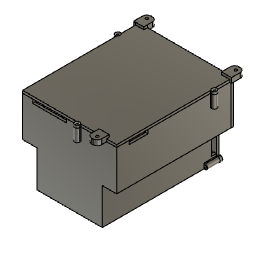
Caja de Circuitos PLA (Autodesk Fusion 360 design; units mm, degrees)
Autodesk Fusion 360 part; units mm, degrees
note: some values were not read from the file. Set by a fixed rule: which sketch regions a step uses.
(part 1 of 2)
sketch "Sketch1" plane through (0, 0, 0) normal (0, 1, 0) x (1, 0, 0)
  line L0 (-24, -14.5) -> (-24, 14.5)
  line L1 (-24, 14.5) -> (24, 14.5)
  line L2 (24, 14.5) -> (24, -14.5)
  line L3 (24, -14.5) -> (-24, 14.5) construction
  line L4 (-24, -14.5) -> (24, 14.5) construction
  line L5 (-24, -14.5) -> (-24, -44.5) construction
  line L6 (-35.5, -44.5) -> (35.5, -44.5) construction
  line L7 (35.5, -44.5) -> (35.5, -14.5)
  line L8 (24, -14.5) -> (-24, -14.5) construction
  line L9 (-35.5, -14.5) -> (-35.5, -44.5)
  line L10 (-35.5, -44.5) -> (35.5, -14.5) construction
  line L11 (35.5, -44.5) -> (-35.5, -14.5) construction
  line L12 (-24, -14.5) -> (-35.5, -14.5)
  line L13 (35.5, -14.5) -> (24, -14.5)
  line L14 (37.5, -44.5) -> (37.5, -12.5)
  line L15 (37.5, -12.5) -> (26, -12.5)
  line L16 (26, 16.5) -> (26, -12.5)
  line L17 (-26, 16.5) -> (26, 16.5)
  line L18 (-26, -12.5) -> (-26, 16.5)
  line L19 (-26, -12.5) -> (-37.5, -12.5)
  line L20 (-37.5, -12.5) -> (-37.5, -44.5)
  line L21 (-37.5, -44.5) -> (-35.5, -44.5)
  line L22 (35.5, -44.5) -> (37.5, -44.5)
  point P0 (0, -29.5)
  dimension "d1" = 48
  dimension "d4" = 29
  dimension "d5" = 30
  dimension "d6" = 71
  dimension "d7" = -2
  constraint parallel L0 L2
  constraint coincident L3 origin
  constraint coincident L4 origin
  constraint horizontal L6
  constraint perpendicular L6 L7
  constraint parallel L6 L8
  constraint parallel L7 L9
  constraint coincident L10 P0
  constraint coincident L11 P0
  constraint parallel L6 L12
  constraint parallel L6 L13
  constraint perpendicular L9 L21
  measures "d1" distance of L0.end L1.end
  measures "d4" distance of L0.start L0.end
  measures "d5" distance of L0.start L5.end
  measures "d6" distance of L7.end L9.start
extrude "Extrude1" add sketch "Sketch1" along normal blind 89 makes body 1
ref_plane "WorkPlane1" through (0, 0, 14) normal (0, -1, 0) x (-1, 0, 0)
sketch "Sketch2" plane through (0, 0, 14) normal (0, -1, 0) x (1, 0, 0)
  line L0 (-37.5, -1.5) -> (-37.5, 30.5)
  line L1 (-26, -1.5) -> (-37.5, -1.5)
  line L2 (-26, -1.5) -> (-26, -30.5)
  line L3 (-26, -30.5) -> (26, -30.5)
  line L4 (26, -30.5) -> (26, -1.5)
  line L5 (37.5, -1.5) -> (26, -1.5)
  line L6 (37.5, 30.5) -> (37.5, -1.5)
  line L7 (-37.5, 30.5) -> (37.5, 30.5)
  constraint coincident L0.end L7.start
  constraint coincident L6.start L7.end
extrude "Extrude2" add sketch "Sketch2" along normal blind 2 bodies 1
ref_plane "WorkPlane2" through (0, 89, 14) normal (0, 1, 0) x (0, 0, 1)
sketch "Sketch3" plane through (0, 89, 14) normal (0, 1, 0) x (1, 0, 0)
  line L0 (-26, 1.5) -> (-26, 30.5)
  line L1 (-26, 30.5) -> (26, 30.5)
  line L2 (26, 30.5) -> (26, 1.5)
  line L3 (26, 1.5) -> (37.5, 1.5)
  line L4 (37.5, 1.5) -> (37.5, -30.5)
  line L5 (37.5, -30.5) -> (-37.5, -30.5)
  line L6 (-37.5, -30.5) -> (-37.5, 1.5)
  line L7 (-37.5, 1.5) -> (-26, 1.5)
extrude "Extrude3" add sketch "Sketch3" along normal blind 2 separate body makes body 2
ref_plane "WorkPlane3" through (0, 43.5, 44.5) normal (0, 0, 1) x (1, 0, 0)
sketch "Sketch4" plane through (0, 43.5, 44.5) normal (0, 0, 1) x (1, 0, 0)
  line L0 (-37.5, 47.5) -> (37.5, 47.5)
  line L1 (-37.5, -45.5) -> (-37.5, 45.5)
  line L2 (37.5, -45.5) -> (-37.5, -45.5)
  line L3 (37.5, -45.5) -> (37.5, 45.5)
  line L4 (-37.5, 45.5) -> (-37.5, 47.5)
  line L5 (37.5, 45.5) -> (37.5, 47.5)
extrude "Extrude4" add sketch "Sketch4" along normal blind 2 bodies 2
ref_plane "WorkPlane4" through (37.5, 43.5, 28.5) normal (1, 0, 0) x (0, 0, -1)
sketch "Sketch5" plane through (37.5, 43.5, 28.5) normal (1, 0, 0) x (0, 1, 0)
  line L0 (-45.5, 16) -> (-35.5, 16) construction
  line L1 (-35.5, 17.9292) -> (-20.5, 17.9292)
  line L2 (-35.5, 16) -> (-20.5, 16)
  line L3 (-20.5, 16) -> (-20.5, 13)
  line L4 (-20.5, 13) -> (-35.5, 13)
  line L5 (-35.5, 13) -> (-35.5, 16)
  point P0 (-45.5, 16)
  dimension "d20" = 10
  dimension "d21" = 15
  dimension "d22" = 3
  constraint coincident P0 L0.start
  constraint horizontal L0
  constraint parallel L0 L1
  constraint horizontal L2
  constraint vertical L3
  constraint horizontal L4
  constraint vertical L5
  measures "d20" distance of P0 L0.end
  measures "d21" distance of L1.start L1.end
  measures "d22" distance of L0.end L4.end
extrude "Extrude5" cut sketch "Sketch5" against normal blind 85 bodies 1
ref_plane "WorkPlane5" through (0, -2, 14) normal (0, -1, 0) x (0, 0, -1)
sketch "Sketch6" plane through (0, -2, 14) normal (0, -1, 0) x (1, 0, 0)
  line L0 (-37.5, 30.5) -> (-29.5, 30.5)
  line L1 (-29.5, 33.204) -> (-2.5, 33.204)
  line L2 (-29.5, 30.5) -> (-2.5, 30.5)
  line L3 (-2.5, 30.5) -> (-2.5, 27.5)
  line L4 (-2.5, 27.5) -> (-29.5, 27.5)
  line L5 (-29.5, 27.5) -> (-29.5, 30.5)
  point P0 (-37.5, 30.5)
  dimension "d26" = 8
  dimension "d27" = 27
  dimension "d28" = 3
  constraint coincident P0 L0.start
  constraint horizontal L0
  constraint parallel L0 L1
  constraint horizontal L2
  constraint vertical L3
  constraint horizontal L4
  constraint vertical L5
  measures "d26" distance of P0 L0.end
  measures "d27" distance of L1.start L1.end
  measures "d28" distance of L0.end L4.end
extrude "Extrude6" cut sketch "Sketch6" against normal blind 10 bodies 1
ref_plane "WorkPlane6" through (0, 43.5, 44.5) normal (0, 0, -1) x (-1, 0, 0)
sketch "Sketch7" plane through (0, 43.5, 44.5) normal (0, 0, -1) x (1, 0, 0)
  line L0 (-37.5, -45.5) -> (37.5, -45.5)
  line L1 (37.5, -45.5) -> (37.5, 45.5)
  line L2 (37.5, 45.5) -> (-37.5, 45.5)
  line L3 (-37.5, 45.5) -> (-37.5, -45.5)
  line L4 (-35.5, -43.5) -> (35.5, -43.5)
  line L5 (35.5, -43.5) -> (35.5, 43.5)
  line L6 (35.5, 43.5) -> (-35.5, 43.5)
  line L7 (-35.5, 43.5) -> (-35.5, -43.5)
  line L8 (-33.5, -41.5) -> (33.5, -41.5)
  line L9 (33.5, -41.5) -> (33.5, 41.5)
  line L10 (33.5, 41.5) -> (-33.5, 41.5)
  line L11 (-33.5, 41.5) -> (-33.5, -41.5)
  line L12 (-29.5, 45.5) -> (-29.5, 41.5)
  line L13 (-2.5, 45.5) -> (-2.5, 41.5)
  line L14 (37.5, 35.5) -> (-35.5, 35.5)
  line L15 (37.5, 20.5) -> (-35.5, 20.5)
  line L16 (-35.5, -41.5) -> (35.5, -41.5)
  point P0 (-29.5, 45.5)
  point P1 (-2.5, 45.5)
  point P2 (37.5, 35.5)
  point P3 (37.5, 20.5)
  dimension "d32" = -2
  dimension "d33" = -4
  constraint coincident P0 L12.start
  constraint coincident L10 L12.end
  constraint perpendicular L10 L12
  constraint coincident P1 L13.start
  constraint coincident L10 L13.end
  constraint perpendicular L10 L13
  constraint coincident P2 L14.start
  constraint coincident L7 L14.end
  constraint perpendicular L7 L14
  constraint coincident P3 L15.start
  constraint coincident L7 L15.end
  constraint perpendicular L7 L15
  constraint coincident L7 L16.start
  constraint coincident L5 L16.end
  constraint perpendicular L5 L16
extrude "Extrude7" add sketch "Sketch7" along normal blind 2 contours L5 L9 L15 L16 | L6 L7 L10 L11 L12 L14 | L5 L6 L9 L10 L13 L14 | L7 L11 L15 L16 bodies 2
ref_plane "WorkPlane7" through (0, 89, 14) normal (0, -1, 0) x (-1, 0, 0)
sketch "Sketch8" plane through (0, 89, 14) normal (0, -1, 0) x (1, 0, 0)
  line L0 (-37.5, 30.5) -> (-37.5, -1.5)
  line L1 (-37.5, -1.5) -> (-26, -1.5)
  line L2 (-26, -1.5) -> (-26, -30.5)
  line L3 (-26, -30.5) -> (26, -30.5)
  line L4 (26, -30.5) -> (26, -1.5)
  line L5 (26, -1.5) -> (37.5, -1.5)
  line L6 (37.5, -1.5) -> (37.5, 30.5)
  line L7 (-35.5, 30.5) -> (-35.5, 0.5)
  line L8 (-35.5, 0.5) -> (-24, 0.5)
  line L9 (-24, 0.5) -> (-24, -28.5)
  line L10 (-24, -28.5) -> (24, -28.5)
  line L11 (24, -28.5) -> (24, 0.5)
  line L12 (24, 0.5) -> (35.5, 0.5)
  line L13 (35.5, 0.5) -> (35.5, 30.5)
  line L14 (-33.5, 30.5) -> (-33.5, 2.5)
  line L15 (-33.5, 2.5) -> (-22, 2.5)
  line L16 (-22, 2.5) -> (-22, -26.5)
  line L17 (-22, -26.5) -> (22, -26.5)
  line L18 (22, -26.5) -> (22, 2.5)
  line L19 (22, 2.5) -> (33.5, 2.5)
  line L20 (33.5, 2.5) -> (33.5, 30.5)
  line L21 (-35.5, 30.5) -> (35.5, 30.5)
  dimension "d37" = -2
  dimension "d38" = -4
  constraint perpendicular L13 L21
extrude "Extrude8" add sketch "Sketch8" along normal blind 2 contours L7 L8 L9 L10 L11 L12 L13 L14 L15 L16 L17 L18 L19 L20 L21 bodies 2
ref_plane "WorkPlane8" through (0, 44.5, 46.5) normal (0, 0, 1) x (1, 0, 0)
sketch "Sketch9" plane through (0, 44.5, 46.5) normal (0, 0, 1) x (1, 0, 0)
  circle A0 centre (7.0001, -47.5) radius 1
  line L0 (8.9999, -46.5) -> (11.0001, -46.5)
  line L1 (8.9999, -46.5) -> (9.0001, -47.4997)
  arc A1 (5.0001, -47.5) -> (9.0001, -47.4997) centre (7.0001, -47.5) ccw
  line L2 (5.0001, -47.5) -> (5.0001, -46.5)
  line L3 (5.0001, -46.5) -> (3.0001, -46.5)
  line L4 (-37.5, -46.5) -> (37.5, -46.5)
  line L5 (35.5, -44.5) -> (-2.5, -44.5)
  line L6 (16.5, -44.5) -> (16.5, -51.9184)
  line L7 (16.5, -51.9184) -> (-2.5, -51.9184)
  line L8 (16.5, -44.5) -> (35.5, -44.5)
  line L9 (26, -44.5) -> (26, -35)
  line L10 (5.0001, -46.5) -> (8.9999, -46.5)
  line L11 (37.5, -21.5) -> (37.5, -36.5)
  line L12 (-37.5, 46.5) -> (-37.5, -46.5)
  line L13 (37.5, -46.5) -> (37.5, 46.5)
  line L14 (37.5, 46.5) -> (-37.5, 46.5)
  line L15 (-37.5, 46.5) -> (-37.5, -46.5)
  line L16 (-37.5, -46.5) -> (37.5, -46.5)
  line L17 (40, -10) -> (-40, -10)
  line L18 (37.5, 32.2975) -> (38.4997, 32.2977)
  arc A2 (38.5, 28.2977) -> (38.4997, 32.2977) centre (38.5, 30.2977) ccw
  line L19 (37.5, 32.2975) -> (37.5, 24.2977)
  line L20 (38.5, 28.2977) -> (37.5, 28.2977)
  circle A3 centre (38.5, 30.2977) radius 1
  line L21 (37.5, 28.2977) -> (37.5, 32.2975)
  line L22 (-38.5, 32.2975) -> (-37.5, 32.2975)
  circle A4 centre (-38.5, 30.2975) radius 1
  arc A5 (-38.5, 32.2975) -> (-38.4997, 28.2975) centre (-38.5, 30.2975) ccw
  line L23 (-37.5, 32.2975) -> (-37.5, 28.2977)
  line L24 (-37.5, 28.2977) -> (-38.4997, 28.2975)
  line L25 (-37.5, 28.2977) -> (-37.5, 16.2975)
  line L26 (37.5, 46.5) -> (33.5003, 46.5)
  line L27 (-33.5003, 46.5) -> (-37.5, 46.5)
  line L28 (-37.5, 30.2976) -> (37.5, 30.2976)
  line L29 (35.4998, 50.5) -> (35.4998, 49.5)
  circle A6 centre (35.4998, 50.5) radius 1
  line L30 (33.4997, 50.5) -> (33.4997, 50.4997)
  arc A7 (33.4997, 50.5) -> (33.4997, 50.4993) centre (35.4998, 50.5) ccw
  arc A8 (38.9998, 50.5) -> (34.9998, 53.9641) centre (35.4998, 50.5) ccw
  line L31 (38.4998, 43.5) -> (37.5, 43.5)
  line L32 (37.5, 46.5) -> (37.5, 43.5)
  line L33 (30.9998, 50.5) -> (30.9998, 46.5)
  line L34 (34.2365, 53.9901) -> (35.7632, 53.9901)
  line L35 (38.9998, 50.5) -> (38.9998, 43.5)
  line L36 (38.9998, 43.5) -> (37.5, 43.5)
  arc A9 (34.9998, 53.9641) -> (30.9998, 50.5) centre (34.4998, 50.5) ccw
  line L37 (0, 46.5) -> (0, 51.2854)
  circle A10 centre (-35.4998, 50.5) radius 1
  line L38 (-33.4997, 50.5) -> (-33.4997, 50.4997)
  line L39 (-30.9998, 50.5) -> (-30.9998, 46.5)
  arc A11 (-34.9998, 53.9641) -> (-38.9998, 50.5) centre (-35.4998, 50.5) ccw
  line L40 (-38.9998, 50.5) -> (-38.9998, 43.5)
  arc A12 (-30.9998, 50.5) -> (-34.9998, 53.9641) centre (-34.4998, 50.5) ccw
  line L41 (-34.2365, 53.9901) -> (-35.7632, 53.9901)
  line L42 (-37.5, 46.5) -> (-33.5003, 46.5)
  line L43 (-37.5, 46.5) -> (-37.5, 43.5)
  line L44 (-35.4998, 50.5) -> (-35.4998, 49.5)
  line L45 (-38.9998, 43.5) -> (-37.5, 43.5)
  arc A13 (-33.4997, 50.4993) -> (-33.4997, 50.5) centre (-35.4998, 50.5) ccw
  line L46 (-38.4998, 43.5) -> (-37.5, 43.5)
  line L47 (26, -49.5) -> (26, -50.5)
  circle A14 centre (26, -50.5) radius 1
  line L48 (21.5, -50.5) -> (21.5, -46.5)
  line L49 (29.5, -50.5) -> (29.5, -46.5)
  line L50 (24.7991, -53.9942) -> (26.1016, -53.9985)
  arc A15 (21.5, -50.5) -> (25.1779, -53.9955) centre (25, -50.5) ccw
  arc A16 (25.9998, -50.5) -> (26, -50.5) centre (26.0002, -48.5) ccw
  arc A17 (25.8753, -53.9978) -> (29.5, -50.5) centre (26, -50.5) ccw
  line L51 (21.5, -46.5) -> (29.5, -46.5)
  point P0 (7.0001, -47.5)
  point P1 (7, -46.5)
  point P2 (26, -46.5)
  point P3 (26.0002, -48.5)
  point P4 (7, -46.5)
  point P5 (37.5, -21.5)
  point P6 (38.5, 30.2977)
  point P7 (37.5, 30.2976)
  point P8 (37.5, 30.2976)
  point P9 (-37.5, 30.2976)
  point P10 (-38.5, 30.2975)
  point P11 (-37.5, 30.2976)
  point P12 (35.5, 48.5)
  point P13 (-37.5, 46.5)
  point P14 (-35.5, 48.5)
  dimension "d42" = 2
  dimension "d2" = 4
  dimension "d48" = 2
  dimension "d49" = 4
  dimension "d50" = 2
  dimension "d51" = 4
  dimension "d128" = 7
  dimension "d129" = 2
  dimension "d135" = 4.5
  constraint coincident A0.centre A1.centre
  constraint concentric A0 A1
  constraint tangent A0 L0
  constraint horizontal L0
  constraint tangent A0 L3
  constraint perpendicular L2 L3
  constraint coincident L1.end A1
  constraint tangent L1 A1
  constraint coincident A1.end L1
  constraint midpoint L5 L6.start
  constraint perpendicular L4 L6
  constraint perpendicular L6 L7
  constraint coincident L5.start L8.end
  constraint midpoint L8 L9.start
  constraint perpendicular L5 L9
  constraint coincident L4 P4
  constraint coincident L4 P2
  constraint parallel L0 L10
  constraint midpoint L10 P4
  constraint perpendicular L15 L17
  constraint coincident P6 A2.centre
  constraint concentric A2 A3
  constraint tangent L19 A3
  constraint coincident L18.end A2
  constraint tangent L18 A2
  constraint coincident A2.end L18
  constraint parallel L19 L21
  constraint midpoint P8 L21
  constraint coincident P10 A4.centre
  constraint concentric A4 A5
  constraint tangent A4 L25
  constraint coincident L24.end A5
  constraint tangent A5 L24
  constraint coincident A5.end L24
  constraint parallel L23 L25
  constraint midpoint P11 L23
  constraint coincident P11 P9
  constraint coincident L13 P8
  constraint perpendicular L13 L28
  constraint vertical L29
  constraint coincident L29.start A6.centre
  constraint concentric A6 A8
  constraint concentric A7 A8
  constraint coincident L13.end L14.start
  constraint coincident L30 A7.end
  constraint coincident L13 L31.end
  constraint perpendicular L13 L31
  constraint coincident L14 L33.end
  constraint perpendicular L14 L33
  constraint coincident A8 L34.end
  constraint perpendicular L33 L34
  constraint tangent A8 L35
  constraint perpendicular L32 L36
  constraint coincident A7 L30.end
  constraint midpoint L14 L37.start
  constraint perpendicular L14 L37
  constraint symmetric L13.end L37 P13
  constraint symmetric P12 L37 P14
  constraint symmetric L26.end L37 L27.start
  constraint symmetric L29.start L37 A10.centre
  constraint symmetric L29.end L37 L44.end
  constraint symmetric A6 L37 A10
  constraint symmetric L30.start L37 L38.start
  constraint symmetric A7 L37 A13
  constraint symmetric A8 L37 A11
  constraint symmetric A7.end L37 A13.start
  constraint symmetric L31.start L37 L46.start
  constraint symmetric L31.end L37 L43.end
  constraint symmetric L33.start L37 L39.start
  constraint symmetric L33.end L37 L39.end
  constraint symmetric L34.start L37 L41.start
  constraint symmetric L34.end L37 L41.end
  constraint symmetric A8.start L37 A11.end
  constraint symmetric L35.end L37 L40.end
  constraint symmetric A9 L37 A12
  constraint symmetric A8.end L37 A11.start
  constraint symmetric L30.end L37 L38.end
  constraint perpendicular L16 L47
  constraint coincident L47.end A14.centre
  constraint concentric A14 A17
  constraint coincident A14 A15.centre
  constraint coincident L4 L48.end
  constraint tangent L48 A15
  constraint coincident L16 L49.end
  constraint tangent L49 A17
  constraint perpendicular L16 L49
  constraint coincident L50.start A15
  constraint coincident L50.end A17
  constraint coincident L50 A15.end
  constraint coincident L50 A17.start
  constraint coincident A14 L47.start
  constraint perpendicular L48 L51
  measures "d42" diameter of A0
  measures "d2" diameter of A1
  measures "d48" diameter of A3
  measures "d49" diameter of A2
  measures "d50" diameter of A4
  measures "d51" diameter of A5
  measures "d128" diameter of A8
  measures "d129" diameter of A6
  measures "d135" distance of L47.end L48.start
extrude "Extrude9" add sketch "Sketch9" against normal blind 2 contours L1 A1 L2 L4 L10 L16 | L12 L15 L22 A5 L23 L24 | L13 L18 A2 L19 L20 L21 bodies 2
ref_plane "WorkPlane9" through (0, 43.5, 44.5) normal (0, 0, 1) x (1, 0, 0)
sketch "Sketch10" plane through (17.5, 3, 44.5) normal (0, 0, 1) x (1, 0, 0)
  circle A0 centre (-56, 71.7975) radius 1
  circle A1 centre (-10.4999, -6) radius 1
  line L0 (-55, 73.7975) -> (-56, 73.7975)
  arc A2 (-56, 73.7975) -> (-55.9997, 69.7975) centre (-56, 71.7975) ccw
  line L1 (-55.9997, 69.7975) -> (-55, 69.7977)
  line L2 (-55, 88) -> (-55, 73.7975)
  line L3 (-8.5001, -5) -> (20, -5)
  line L4 (-12.4999, -5) -> (-12.4999, -6)
  arc A3 (-12.4999, -6) -> (-8.4999, -5.9997) centre (-10.4999, -6) ccw
  line L5 (-8.4999, -5.9997) -> (-8.5001, -5)
  line L6 (20, 73.7975) -> (20, 88)
  line L7 (20, 88) -> (-55, 88)
  line L8 (-12.4999, -5) -> (-8.5001, -5)
  line L9 (-55, 88) -> (-55, 73.7975)
  circle A4 centre (21, 71.7977) radius 1
  line L10 (20, 69.7977) -> (21, 69.7977)
  arc A5 (21, 69.7977) -> (20.9997, 73.7977) centre (21, 71.7977) ccw
  line L11 (20.9997, 73.7977) -> (20, 73.7975)
  line L12 (20, -5) -> (20, 69.7977)
  line L13 (20, 73.7975) -> (20, 69.7977)
  line L14 (20, 73.7975) -> (20, 69.7977)
  line L15 (-55, 69.7977) -> (-55, -5)
  line L16 (-55, -5) -> (-12.4999, -5)
  constraint coincident L4.start L8.start
  constraint coincident L3.start L5.end
  constraint coincident L2.start L7.end
  constraint coincident L0.start L2.end
  constraint coincident L6.start L11.end
  constraint coincident L10.start L12.end
extrude "Extrude11" add sketch "Sketch10" against normal blind 10 bodies 1
fillet "Fillet1" radius 0.95 3 edges at (6.0678, -3.3616, 46.5) (37.5677, 74.4361, 46.5) (-39.4323, 74.4359, 46.5) on bodies 2
ref_plane "WorkPlane10" through (0, 91, 15) normal (0, 1, 0) x (0, 0, 1)
sketch "Sketch11" plane through (0, 91, 15) normal (0, 1, 0) x (1, 0, 0)
  line L0 (26, 31.5) -> (26, 33.5002)
  line L1 (26, 27.5002) -> (26, 25.5002)
  line L2 (26, 31.5) -> (26.9997, 31.5002)
  circle A0 centre (27, 29.5002) radius 1
  line L3 (27, 27.5002) -> (26, 27.5002)
  arc A1 (27, 27.5002) -> (26.9997, 31.5002) centre (27, 29.5002) ccw
  line L4 (-26, 27.5002) -> (-26, 25.5)
  line L5 (-26, 31.5) -> (-26, 33.5)
  line L6 (-26, 27.5002) -> (-26.9997, 27.5)
  arc A2 (-27, 31.5) -> (-26.9997, 27.5) centre (-27, 29.5) ccw
  circle A3 centre (-27, 29.5) radius 1
  line L7 (-27, 31.5) -> (-26, 31.5)
  line L8 (37.5, -31.5) -> (37.5, 2.5)
  line L9 (37.5, 2.5) -> (26, 2.5)
  line L10 (26, 2.5) -> (26, 31.5)
  line L11 (26, 31.5) -> (-26, 31.5)
  line L12 (-26, 31.5) -> (-26, 2.5)
  line L13 (-26, 2.5) -> (-37.5, 2.5)
  line L14 (-37.5, 2.5) -> (-37.5, -31.5)
  line L15 (-37.5, -31.5) -> (37.5, -31.5)
  line L16 (26, 27.5002) -> (26, 31.5)
  line L17 (-26, 27.5002) -> (-26, 31.5)
  point P0 (27, 29.5002)
  point P1 (-27, 29.5)
  dimension "d64" = 2
  dimension "d65" = 4
  dimension "d66" = 2
  dimension "d67" = 4
  constraint coincident P0 A0.centre
  constraint concentric A0 A1
  constraint tangent L0 A0
  constraint tangent L1 A0
  constraint perpendicular L1 L3
  constraint coincident L2.end A1
  constraint tangent L2 A1
  constraint coincident A1.end L2
  constraint coincident P1 A2.centre
  constraint concentric A2 A3
  constraint tangent L4 A3
  constraint tangent L5 A3
  constraint perpendicular L5 L7
  constraint coincident L6.end A2
  constraint tangent L6 A2
  constraint coincident A2.end L6
  constraint parallel L0 L16
  constraint parallel L4 L17
  measures "d64" diameter of A0
  measures "d65" diameter of A1
  measures "d66" diameter of A3
  measures "d67" diameter of A2
extrude "Extrude12" add sketch "Sketch11" against normal blind 2 contours L2 L3 A1 L10 L16 | L6 A2 L7 L12 L17 bodies 2
ref_plane "WorkPlane11" through (0, 89, 14) normal (0, 1, 0) x (0, 0, 1)
sketch "Sketch12" plane through (0, 89, 14) normal (0, 1, 0) x (1, 0, 0)
  circle A0 centre (27, 28.5002) radius 1
  line L0 (26, 26.5002) -> (27, 26.5002)
  arc A1 (27, 26.5002) -> (26.9997, 30.5002) centre (27, 28.5002) ccw
  line L1 (26.9997, 30.5002) -> (26, 30.5)
  line L2 (26, 30.5) -> (-27, 30.5)
  arc A2 (-27, 30.5) -> (-26.9997, 26.5) centre (-27, 28.5) ccw
  line L3 (-26.9997, 26.5) -> (-26, 26.5002)
  line L4 (-26, 26.5002) -> (-26, 1.5)
  line L5 (-26, 1.5) -> (-37.5, 1.5)
  line L6 (-37.5, 1.5) -> (-37.5, -32.5)
  line L7 (-37.5, -32.5) -> (37.5, -32.5)
  line L8 (37.5, -32.5) -> (37.5, 1.5)
  line L9 (37.5, 1.5) -> (26, 1.5)
  line L10 (26, 1.5) -> (26, 26.5002)
  circle A3 centre (-27, 28.5) radius 1
  line L11 (-26, 26.5002) -> (-26, 30.5)
  line L12 (26, 26.5002) -> (26, 30.5)
  constraint coincident L3.end L4.start
  constraint coincident L2 L11.end
  constraint perpendicular L2 L11
  constraint coincident L0.start L10.end
  constraint coincident L1.end L2.start
extrude "Extrude13" add sketch "Sketch12" against normal blind 10 contours L0 A1 L1 L12 | L2 A2 L3 L11 bodies 1
fillet "Fillet2" radius 0.75 1 edges at (26.0677, 91, -14.1386) on bodies 2
fillet "Fillet3" radius 0.75 1 edges at (-27.9323, 91, -14.1384) on bodies 2
ref_plane "WorkPlane12" through (0, 42.8453, 46.5) normal (0, 0, 1) x (1, 0, 0)
sketch "Sketch13" plane through (0, 44.5, 46.5) normal (0, 0, 1) x (1, 0, 0)
  line L0 (22.8485, -17.0341) -> (42.8485, -17.0341)
  line L1 (30.8608, -5.5292) -> (30.8608, -9.5292)
  line L2 (31.1608, 9.1708) -> (34.5608, 9.1708)
  line L3 (30.8608, 5.4708) -> (34.8608, 5.4708)
  line L4 (42.8485, 0.9659) -> (42.8485, 15.9659)
  circle A0 centre (32.8608, -7.5292) radius 3.5
  line L5 (34.5608, 9.1708) -> (34.5608, 5.7708)
  line L6 (38.8608, 13.4708) -> (26.8608, 13.4708)
  line L7 (34.8608, -5.5292) -> (30.8608, -5.5292)
  line L8 (34.5608, -5.8292) -> (34.5608, -9.2292)
  line L9 (38.8608, 1.4708) -> (38.8608, 13.4708)
  line L10 (34.8608, 5.4708) -> (34.8608, 9.4708)
  line L11 (-43.0733, -15.704) -> (-23.0733, -15.704)
  spline S0 degree 3 poles (55.2858, -54.3578) (54.3358, -55.3128) (53.3125, -56.2332) (48.6473, -59.3219) (45.227, -60.7727) (34.4807, -63.8175) (26.4794, -64.594) (11.0534, -65.2226) (3.7466, -65.1878) (-14.555, -65.1533) (-25.3526, -64.9716) (-38.807, -62.6517) (-43.1147, -61.5744) (-48.6935, -59.1167) (-50.3493, -58.2272) (-53.373, -56.1542) (-54.405, -55.2432) (-55.2858, -54.3578) knots 0.099374 0.099374 0.099374 0.099374 0.511391 0.511391 1.184373 1.184373 2.365156 2.365156 3.424834 3.424834 5.021087 5.021087 5.733233 5.733233 6.048425 6.048425 6.350752 6.350752 6.350752 6.350752
  circle A1 centre (-18.4548, -24.5744) radius 4
  line L12 (2, -22.4518) -> (2, -24.4591)
  line L13 (-2, -24.4591) -> (-2, -22.4518)
  line L14 (-39.3583, -13.4184) -> (-27.3583, -13.4184)
  spline S1 degree 3 poles (-57.4133, -56.4733) (-54.6548, -59.2461) (-51.3263, -61.286) (-43.7762, -64.4978) (-39.4461, -65.5832) (-26.1242, -67.8896) (-15.7362, -68.1341) (-2.1162, -68.1815) (3.28, -68.1844) (16.6163, -68.1041) (26.1936, -67.8222) (40.0568, -65.5096) (45.0142, -64.1652) (52.3092, -60.6607) (55.0683, -58.8304) (57.4133, -56.4733) knots -11.261923 -11.261923 -11.261923 -11.261923 -9.981891 -9.981891 -8.573851 -8.573851 -5.544519 -5.544519 -4.707919 -4.707919 -2.429331 -2.429331 -0.997479 -0.997479 0 0 0 0
  line L15 (-23.0733, -15.704) -> (-23.0733, 17.296)
  circle A2 centre (7.4393, 32.9811) radius 3.5
  line L16 (5.4393, 34.9811) -> (5.4393, 30.9811)
  line L17 (13.4393, 26.9811) -> (13.4393, 38.9811)
  line L18 (1.4393, 38.9811) -> (1.4393, 26.9811)
  line L19 (9.1393, 31.2811) -> (5.7393, 31.2811)
  circle A3 centre (7.4393, 32.9811) radius 3.5
  line L20 (13.4393, 38.9811) -> (1.4393, 38.9811)
  line L21 (-1.5607, 26.9811) -> (-1.5607, 38.9811)
  line L22 (1.4393, 26.9811) -> (13.4393, 26.9811)
  line L23 (17.3207, 23.0477) -> (17.3207, 43.0477)
  line L24 (17.3207, 43.0477) -> (-0.6793, 43.0477)
  line L25 (5.7393, 31.2811) -> (5.7393, 34.6811)
  line L26 (5.7393, 34.6811) -> (9.1393, 34.6811)
  circle A4 centre (7.4393, 32.9811) radius 3.5
  line L27 (9.1393, 34.6811) -> (9.1393, 31.2811)
  line L28 (38.8608, -13.5292) -> (38.8608, -1.5292)
  line L29 (30.8608, 9.4708) -> (30.8608, 5.4708)
  line L30 (31.1608, 5.7708) -> (31.1608, 9.1708)
  line L31 (31.1608, -9.2292) -> (31.1608, -5.8292)
  line L32 (34.8608, 9.4708) -> (30.8608, 9.4708)
  line L33 (38.8608, -1.5292) -> (26.8608, -1.5292)
  line L34 (30.8608, -9.5292) -> (34.8608, -9.5292)
  line L35 (26.8608, 1.4708) -> (38.8608, 1.4708)
  line L36 (26.8608, 13.4708) -> (26.8608, 1.4708)
  line L37 (34.5608, 5.7708) -> (31.1608, 5.7708)
  line L38 (34.5608, -9.2292) -> (31.1608, -9.2292)
  line L39 (34.8608, -9.5292) -> (34.8608, -5.5292)
  line L40 (42.8485, 15.9659) -> (22.8485, 15.9659)
  circle A5 centre (32.8608, -7.5292) radius 3.5
  circle A6 centre (32.8608, 7.4708) radius 3.5
  line L41 (31.1608, -5.8292) -> (34.5608, -5.8292)
  circle A7 centre (-7.5607, 32.9811) radius 3.5
  line L42 (-9.2607, 34.6811) -> (-5.8607, 34.6811)
  line L43 (-5.5607, 30.9811) -> (-5.5607, 34.9811)
  line L44 (-5.5607, 34.9811) -> (-9.5607, 34.9811)
  line L45 (-5.8607, 34.6811) -> (-5.8607, 31.2811)
  line L46 (34.8608, 5.4708) -> (34.8608, 9.4708)
  line L47 (-13.5607, 38.9811) -> (-13.5607, 26.9811)
  circle A8 centre (32.8608, 7.4708) radius 3.5
  line L48 (26.8608, -13.5292) -> (38.8608, -13.5292)
  circle A9 centre (32.8608, 7.4708) radius 3.5
  circle A10 centre (32.8608, -7.5292) radius 3.5
  arc A11 (2, -24.4591) -> (-2, -24.4591) centre (0, -0.0409) ccw
  circle A12 centre (-33.3583, -7.4184) radius 3.5
  spline S2 degree 3 poles (57.4133, -56.4733) (60.1938, -53.6783) (62.232, -50.3026) (65.4397, -42.6602) (66.5242, -38.2667) (68.8286, -24.7614) (69.073, -14.2254) (69.1297, 2.6103) (69.126, 11.9307) (68.7296, 23.9203) (68.3137, 30.2773) (66.4441, 41.6398) (65.0937, 46.6797) (61.5854, 54.0505) (59.7633, 56.8293) (57.4133, 59.1915) knots -11.16303 -11.16303 -11.16303 -11.16303 -9.933997 -9.933997 -8.576307 -8.576307 -5.651579 -5.651579 -4.027278 -4.027278 -2.4504 -2.4504 -0.99962 -0.99962 0 0 0 0
  arc A13 (2, -22.4518) -> (-2, -22.4518) centre (0, -0.0409) ccw
  line L49 (-35.3583, -9.4184) -> (-31.3583, -9.4184)
  line L50 (-35.3583, 9.5816) -> (-35.3583, 5.5816)
  line L51 (-13.5607, 26.9811) -> (-1.5607, 26.9811)
  circle A14 centre (-33.3583, -7.4184) radius 3.5
  line L52 (-31.3583, -9.4184) -> (-31.3583, -5.4184)
  line L53 (22.8485, 15.9659) -> (22.8485, -17.0341)
  line L54 (-9.2607, 31.2811) -> (-9.2607, 34.6811)
  line L55 (42.8485, -17.0341) -> (42.8485, 0.9659)
  circle A15 centre (-33.3583, 7.5816) radius 3.5
  line L56 (-5.8607, 31.2811) -> (-9.2607, 31.2811)
  circle A16 centre (-7.5607, 32.9811) radius 3.5
  line L57 (-31.6583, -9.1184) -> (-35.0583, -9.1184)
  line L58 (-23.0733, 17.296) -> (-43.0733, 17.296)
  line L59 (-31.3583, 5.5816) -> (-31.3583, 9.5816)
  line L60 (-0.6793, 43.0477) -> (-15.6793, 43.0477)
  circle A17 centre (0.1301, 0.0814) radius 15
  line L61 (-27.3583, -13.4184) -> (-27.3583, -1.4184)
  circle A18 centre (0.1339, -0.0943) radius 20.7403
  spline S3 degree 3 poles (55.2858, 57.0761) (57.3948, 54.9561) (59.0247, 52.4489) (62.2615, 45.649) (63.5323, 40.8577) (65.546, 28.6194) (65.9265, 20.7301) (66.1452, 6.6494) (66.1342, -2.4184) (65.9854, -17.2205) (65.6015, -26.8325) (63.2719, -38.8883) (62.2402, -42.7062) (59.3648, -49.1939) (57.6185, -52.013) (55.2858, -54.3578) knots 0 0 0 0 0.897083 0.897083 2.263855 2.263855 4.144612 4.144612 5.50519 5.50519 8.112257 8.112257 9.275061 9.275061 10.285153 10.285153 10.285153 10.285153
  line L62 (-43.0733, -0.704) -> (-43.0733, -15.704)
  line L63 (-15.6793, 23.0477) -> (17.3207, 23.0477)
  line L64 (-35.0583, 5.8816) -> (-35.0583, 9.2816)
  line L65 (-43.0733, 17.296) -> (-43.0733, -0.704)
  line L66 (-9.5607, 34.9811) -> (-9.5607, 30.9811)
  line L67 (-35.0583, 9.2816) -> (-31.6583, 9.2816)
  circle A19 centre (-33.3583, 7.5816) radius 3.5
  line L68 (-31.3583, -5.4184) -> (-35.3583, -5.4184)
  line L69 (-35.3583, 5.5816) -> (-31.3583, 5.5816)
  line L70 (-35.0583, -9.1184) -> (-35.0583, -5.7184)
  line L71 (-39.3583, 13.5816) -> (-39.3583, 1.5816)
  line L72 (-35.0583, -5.7184) -> (-31.6583, -5.7184)
  line L73 (26.8608, -1.5292) -> (26.8608, -13.5292)
  line L74 (-31.6583, -5.7184) -> (-31.6583, -9.1184)
  line L75 (-9.5607, 30.9811) -> (-5.5607, 30.9811)
  line L76 (-31.3583, 9.5816) -> (-35.3583, 9.5816)
  line L77 (-27.3583, -1.4184) -> (-39.3583, -1.4184)
  line L78 (-35.3583, -5.4184) -> (-35.3583, -9.4184)
  line L79 (-39.3583, 1.5816) -> (-27.3583, 1.5816)
  circle A20 centre (-7.5607, 32.9811) radius 3.5
  line L80 (-1.5607, 38.9811) -> (-13.5607, 38.9811)
  line L81 (-27.3583, 1.5816) -> (-27.3583, 13.5816)
  spline S4 degree 3 poles (-55.2858, 57.0761) (-54.3358, 58.031) (-53.3125, 58.9514) (-48.6473, 62.0401) (-45.227, 63.4909) (-34.4807, 66.5357) (-26.4794, 67.3122) (-11.0534, 67.9408) (-3.7466, 67.906) (14.555, 67.8716) (25.3526, 67.6898) (38.807, 65.37) (43.1147, 64.2926) (48.6935, 61.835) (50.3493, 60.9455) (53.373, 58.8725) (54.405, 57.9614) (55.2858, 57.0761) knots 0.099374 0.099374 0.099374 0.099374 0.511391 0.511391 1.184373 1.184373 2.365156 2.365156 3.424834 3.424834 5.021087 5.021087 5.733233 5.733233 6.048425 6.048425 6.350752 6.350752 6.350752 6.350752
  spline S5 degree 3 poles (57.4133, 59.1915) (56.0007, 60.6114) (54.4331, 61.8451) (50.9868, 64.0379) (49.1171, 64.9721) (42.9907, 67.4743) (38.3806, 68.5462) (24.2455, 70.7699) (13.2443, 70.8871) (-14.7495, 70.9078) (-24.9972, 70.74) (-40.0568, 68.2279) (-45.0142, 66.8834) (-52.3092, 63.3789) (-55.0683, 61.5487) (-57.4133, 59.1915) knots -8.304429 -8.304429 -8.304429 -8.304429 -7.948055 -7.948055 -7.577573 -7.577573 -6.770175 -6.770175 -5.028128 -5.028128 -2.429331 -2.429331 -0.997479 -0.997479 0 0 0 0
  circle A21 centre (-33.3583, 7.5816) radius 3.5
  spline S6 degree 3 poles (-55.2858, -54.3578) (-57.3948, -52.2379) (-59.0247, -49.7307) (-62.2615, -42.9308) (-63.5323, -38.1395) (-65.546, -25.9012) (-65.9265, -18.0119) (-66.1452, -3.9311) (-66.1342, 5.1367) (-65.9854, 19.9388) (-65.6015, 29.5508) (-63.2719, 41.6065) (-62.2402, 45.4245) (-59.3648, 51.9121) (-57.6185, 54.7312) (-55.2858, 57.0761) knots 0 0 0 0 0.897083 0.897083 2.263855 2.263855 4.144613 4.144613 5.50519 5.50519 8.112254 8.112254 9.275057 9.275057 10.285148 10.285148 10.285148 10.285148
  circle A22 centre (0.1339, -0.0943) radius 22
  spline S7 degree 3 poles (-57.4133, 59.1915) (-60.0163, 56.575) (-61.9697, 53.4489) (-65.0965, 46.3744) (-66.1916, 42.3341) (-68.6024, 29.7801) (-68.9894, 19.9785) (-69.1331, 5.0405) (-69.1463, -4.156) (-68.9151, -18.3795) (-68.5208, -26.3005) (-66.4441, -38.9215) (-65.0937, -43.9615) (-61.5854, -51.3322) (-59.7633, -54.111) (-57.4133, -56.4733) knots -11.000258 -11.000258 -11.000258 -11.000258 -9.829581 -9.829581 -8.544746 -8.544746 -5.760766 -5.760766 -4.36264 -4.36264 -2.4504 -2.4504 -0.99962 -0.99962 0 0 0 0
  line L82 (-15.6793, 43.0477) -> (-15.6793, 23.0477)
  line L83 (-31.6583, 9.2816) -> (-31.6583, 5.8816)
  line L84 (-39.3583, -1.4184) -> (-39.3583, -13.4184)
  circle A23 centre (0.1339, -0.0943) radius 15.5
  circle A24 centre (0.1339, 0.4057) radius 20.7403
  circle A25 centre (0.1339, 0.4057) radius 16.5
  circle A26 centre (-33.3583, -7.4184) radius 3.5
  line L85 (-27.3583, 13.5816) -> (-39.3583, 13.5816)
  line L86 (-31.6583, 5.8816) -> (-35.0583, 5.8816)
  circle A27 centre (-18.4548, -24.5744) radius 4.5
  line L87 (-10.0984, -23.101) -> (-19.9283, -16.2181)
  line L88 (-19.9283, -16.2181) -> (-26.8112, -26.0479)
  line L89 (-26.8112, -26.0479) -> (-16.9814, -32.9308)
  line L90 (-16.9814, -32.9308) -> (-10.0984, -23.101)
  line L91 (-10.0984, -23.101) -> (-26.8112, -26.0479) construction
  line L92 (-19.9283, -16.2181) -> (-16.9814, -32.9308) construction
  line L93 (9.906, -23.2119) -> (16.7889, -33.0418)
  line L94 (16.7889, -33.0418) -> (26.6188, -26.1589)
  line L95 (26.6188, -26.1589) -> (19.7359, -16.329)
  line L96 (19.7359, -16.329) -> (9.906, -23.2119)
  line L97 (9.906, -23.2119) -> (26.6188, -26.1589) construction
  line L98 (19.7359, -16.329) -> (16.7889, -33.0418) construction
  circle A28 centre (18.2624, -24.6854) radius 4.5
  circle A29 centre (18.2624, -24.6854) radius 4
  line L99 (-5.892, -24.5492) -> (-5.892, -36.5492)
  line L100 (-5.892, -36.5492) -> (6.108, -36.5492)
  line L101 (6.108, -36.5492) -> (6.108, -24.5492)
  line L102 (6.108, -24.5492) -> (-5.892, -24.5492)
  line L103 (-5.892, -24.5492) -> (6.108, -36.5492) construction
  line L104 (6.108, -24.5492) -> (-5.892, -36.5492) construction
  circle A30 centre (0.108, -30.5492) radius 4.5
  circle A31 centre (0.108, -30.5492) radius 4
  circle A32 centre (38.5, 30.2977) radius 1.95
  line L105 (37.5, 28.2977) -> (38.5, 28.2977)
  arc A33 (38.5, 28.2977) -> (38.4997, 32.2977) centre (38.5, 30.2977) ccw
  line L106 (38.4997, 32.2977) -> (37.5, 32.2975)
  line L107 (37.5, 32.2975) -> (37.5, 46.5)
  line L108 (37.5, 46.5) -> (-37.5, 46.5)
  line L109 (-37.5, 46.5) -> (-37.5, 32.2975)
  line L110 (-37.5, 32.2975) -> (-38.5, 32.2975)
  arc A34 (-38.5, 32.2975) -> (-38.4997, 28.2975) centre (-38.5, 30.2975) ccw
  line L111 (-38.4997, 28.2975) -> (-37.5, 28.2977)
  line L112 (-37.5, 28.2977) -> (-37.5, -46.5)
  line L113 (8.9999, -46.5) -> (37.5, -46.5)
  line L114 (5.0001, -46.5) -> (5.0001, -47.5)
  arc A35 (5.0001, -47.5) -> (9.0001, -47.4997) centre (7.0001, -47.5) ccw
  line L115 (9.0001, -47.4997) -> (8.9999, -46.5)
  line L116 (37.5, -46.5) -> (37.5, 28.2977)
  circle A36 centre (7.0001, -47.5) radius 1.95
  circle A37 centre (-38.5, 30.2975) radius 1.95
  line L117 (37.5, -46.5) -> (37.5, -53.3896)
  line L118 (26.0003, -50.5) -> (39, -50.5)
  line L119 (-37.5007, 50.5) -> (37.5, 50.5)
  line L120 (37.5, 50.5) -> (37.5, -50.5)
  line L121 (37.5, -50.5) -> (-37.5007, -50.5)
  line L122 (-37.5007, -50.5) -> (-37.5007, 50.5)
  line L123 (-37.5, -46.5) -> (5.0001, -46.5)
  point P0 (-18.4548, -24.5744)
  point P1 (26.0003, -50.5)
  point P2 (-35.5005, 50.5)
  dimension "d78" = 9
  dimension "d81" = 12
  dimension "d82" = 12
  dimension "d83" = 9
  dimension "d84" = 12
  dimension "d85" = 12
  dimension "d86" = 9
  dimension "d87" = 12
  dimension "d88" = 12
  constraint concentric A1 A27
  constraint perpendicular L87 L88
  constraint parallel L87 L89
  constraint parallel L88 L90
  constraint coincident L91 P0
  constraint coincident L92 P0
  constraint coincident P0 A1.centre
  constraint concentric A28 A29
  constraint perpendicular L93 L96
  constraint parallel L94 L96
  constraint parallel L93 L95
  constraint concentric A30 A31
  constraint perpendicular L99 L102
  constraint parallel L100 L102
  constraint parallel L99 L101
  constraint coincident L113.end L116.start
  constraint coincident P1 L118.start
  constraint perpendicular L117 L118
  constraint horizontal L119
  constraint vertical L120
  constraint horizontal L121
  constraint vertical L122
  constraint coincident L117 L120.end
  constraint coincident L118 L120.end
  measures "d78" diameter of A27
  measures "d81" distance of L88.end L89.end
  measures "d82" distance of L87.end L88.end
  measures "d83" diameter of A28
  measures "d84" distance of L93.end L94.end
  measures "d85" distance of L93.start L93.end
  measures "d86" diameter of A30
  measures "d87" distance of L99.end L100.end
  measures "d88" distance of L99.start L99.end
ref_plane "WorkPlane13" through (0.1301, 44.5814, 46.5) normal (0, 0, 1) x (1, 0, 0)
sketch "Sketch14" plane through (0.1301, 44.5814, 46.5) normal (0, 0, 1) x (1, 0, 0)
  circle A0 centre (0, 0.9) radius 64
  spline S0 degree 3 poles (55.1557, 56.9947) (57.2647, 54.8747) (58.8946, 52.3676) (62.1314, 45.5676) (63.4022, 40.7763) (65.416, 28.5381) (65.7964, 20.6488) (66.0151, 6.568) (66.0041, -2.4998) (65.8553, -17.3019) (65.4714, -26.9139) (63.1418, -38.9696) (62.1101, -42.7876) (59.2348, -49.2752) (57.4884, -52.0943) (55.1557, -54.4392) knots 0 0 0 0 0.897083 0.897083 2.263855 2.263855 4.144612 4.144612 5.50519 5.50519 8.112257 8.112257 9.275061 9.275061 10.285153 10.285153 10.285153 10.285153
  spline S1 degree 3 poles (57.2832, -56.5546) (60.0637, -53.7597) (62.1019, -50.384) (65.3096, -42.7416) (66.3941, -38.3481) (68.6985, -24.8428) (68.9429, -14.3068) (68.9996, 2.5289) (68.9959, 11.8493) (68.5995, 23.839) (68.1836, 30.1959) (66.314, 41.5584) (64.9636, 46.5983) (61.4553, 53.9691) (59.6332, 56.7479) (57.2832, 59.1101) knots -11.16303 -11.16303 -11.16303 -11.16303 -9.933997 -9.933997 -8.576307 -8.576307 -5.651579 -5.651579 -4.027278 -4.027278 -2.4504 -2.4504 -0.99962 -0.99962 0 0 0 0
  spline S2 degree 3 poles (-55.4159, 56.9947) (-54.4659, 57.9496) (-53.4426, 58.87) (-48.7774, 61.9587) (-45.3571, 63.4096) (-34.6108, 66.4544) (-26.6095, 67.2309) (-11.1835, 67.8595) (-3.8767, 67.8246) (14.4249, 67.7902) (25.2226, 67.6085) (38.6769, 65.2886) (42.9846, 64.2112) (48.5634, 61.7536) (50.2192, 60.8641) (53.2429, 58.7911) (54.2749, 57.8801) (55.1557, 56.9947) knots 0.099374 0.099374 0.099374 0.099374 0.511391 0.511391 1.184373 1.184373 2.365156 2.365156 3.424834 3.424834 5.021087 5.021087 5.733233 5.733233 6.048425 6.048425 6.350752 6.350752 6.350752 6.350752
  spline S3 degree 3 poles (57.2832, 59.1101) (55.8706, 60.5301) (54.3031, 61.7637) (50.8567, 63.9566) (48.987, 64.8907) (42.8606, 67.3929) (38.2505, 68.4648) (24.1154, 70.6885) (13.1142, 70.8057) (-14.8796, 70.8264) (-25.1273, 70.6587) (-40.1869, 68.1465) (-45.1443, 66.8021) (-52.4393, 63.2976) (-55.1984, 61.4673) (-57.5434, 59.1101) knots -8.304429 -8.304429 -8.304429 -8.304429 -7.948055 -7.948055 -7.577573 -7.577573 -6.770175 -6.770175 -5.028128 -5.028128 -2.429331 -2.429331 -0.997479 -0.997479 0 0 0 0
  spline S4 degree 3 poles (-55.4159, -54.4392) (-57.5249, -52.3193) (-59.1548, -49.8121) (-62.3916, -43.0121) (-63.6624, -38.2208) (-65.6761, -25.9826) (-66.0565, -18.0933) (-66.2753, -4.0125) (-66.2643, 5.0553) (-66.1155, 19.8574) (-65.7316, 29.4694) (-63.402, 41.5251) (-62.3703, 45.3431) (-59.4949, 51.8307) (-57.7486, 54.6498) (-55.4159, 56.9947) knots 0 0 0 0 0.897083 0.897083 2.263855 2.263855 4.144613 4.144613 5.50519 5.50519 8.112254 8.112254 9.275057 9.275057 10.285148 10.285148 10.285148 10.285148
  spline S5 degree 3 poles (-57.5434, 59.1101) (-60.1464, 56.4936) (-62.0998, 53.3675) (-65.2266, 46.2931) (-66.3217, 42.2527) (-68.7325, 29.6987) (-69.1194, 19.8971) (-69.2632, 4.9591) (-69.2764, -4.2374) (-69.0452, -18.4609) (-68.6509, -26.3819) (-66.5741, -39.0029) (-65.2238, -44.0428) (-61.7155, -51.4136) (-59.8934, -54.1924) (-57.5434, -56.5546) knots -11.000258 -11.000258 -11.000258 -11.000258 -9.829581 -9.829581 -8.544746 -8.544746 -5.760766 -5.760766 -4.36264 -4.36264 -2.4504 -2.4504 -0.99962 -0.99962 0 0 0 0
  spline S6 degree 3 poles (-57.5434, -56.5546) (-54.7849, -59.3275) (-51.4564, -61.3674) (-43.9063, -64.5792) (-39.5762, -65.6646) (-26.2543, -67.971) (-15.8663, -68.2155) (-2.2463, -68.2629) (3.15, -68.2658) (16.4862, -68.1854) (26.0635, -67.9036) (39.9267, -65.591) (44.8841, -64.2466) (52.1792, -60.7421) (54.9382, -58.9118) (57.2832, -56.5546) knots -11.261923 -11.261923 -11.261923 -11.261923 -9.981891 -9.981891 -8.573851 -8.573851 -5.544519 -5.544519 -4.707919 -4.707919 -2.429331 -2.429331 -0.997479 -0.997479 0 0 0 0
  spline S7 degree 3 poles (55.1557, -54.4392) (54.2057, -55.3942) (53.1824, -56.3145) (48.5172, -59.4033) (45.0969, -60.8541) (34.3506, -63.8989) (26.3493, -64.6754) (10.9233, -65.304) (3.6165, -65.2692) (-14.6851, -65.2347) (-25.4827, -65.053) (-38.9371, -62.7331) (-43.2448, -61.6557) (-48.8236, -59.1981) (-50.4794, -58.3086) (-53.5031, -56.2356) (-54.5351, -55.3246) (-55.4159, -54.4392) knots 0.099374 0.099374 0.099374 0.099374 0.511391 0.511391 1.184373 1.184373 2.365156 2.365156 3.424834 3.424834 5.021087 5.021087 5.733233 5.733233 6.048425 6.048425 6.350752 6.350752 6.350752 6.350752
  dimension "d91" = 128
  measures "d91" diameter of A0
ref_plane "WorkPlane16" through (0, -2, 14) normal (0, -1, 0) x (0, 0, -1)
sketch "Sketch16" plane through (0, -2, 14) normal (0, -1, 0) x (1, 0, 0)
  line L0 (5, 32.5) -> (5, 62.5)
  line L1 (-4, -30.5) -> (-4, 32.5)
  line L2 (-59.178, -30.5) -> (-59.178, 41.5)
  line L3 (-4, 32.5) -> (-70, 32.5)
  line L4 (-59.178, 41.5) -> (60, 41.5)
  line L5 (-59.178, 41.5) -> (-59.178, 62.5)
  line L6 (-59.178, 62.5) -> (60, 62.5)
  dimension "d95" = 30
  dimension "d96" = 63
  dimension "d97" = 72
  dimension "d98" = 21
  constraint vertical L0
  constraint vertical L1
  constraint parallel L1 L2
  constraint perpendicular L1 L3
  constraint perpendicular L2 L4
  constraint perpendicular L4 L5
  constraint perpendicular L0 L6
  measures "d95" distance of L0.start L0.end
  measures "d96" distance of L1.start L1.end
  measures "d97" distance of L2.start L2.end
  measures "d98" distance of L2.end L5.end
ref_plane "WorkPlane17" through (0, 45, 0) normal (0, 1, 0) x (0, 0, 1)
sketch "Sketch17" plane through (0, 45, 0) normal (0, 1, 0) x (1, 0, 0)
  line L0 (19.1369, -77.5) -> (-0.3631, -77.5)
  line L1 (63.7288, -50) -> (-63.7288, -50)
  line L2 (19.1369, -77.5) -> (19.1369, -50)
  dimension "d101" = 27.5
  constraint coincident L0.start L2.start
  constraint coincident L1 L2.end
  constraint perpendicular L1 L2
  measures "d101" distance of L0.start L2.end
ref_plane "WorkPlane18" through (0, 0, 120) normal (0, 0, 1) x (1, 0, 0)
sketch "Sketch18" plane through (0, 0, 120) normal (0, 0, 1) x (1, 0, 0)
  line L0 (-0.3631, 88.6361) -> (-0.3631, 90.1361)
  line L1 (-0.3631, 90.1361) -> (-15.3631, 90.1361)
  line L2 (-15.3631, 90.1361) -> (-15.3631, 68.4361)
  line L3 (-15.3631, 68.4361) -> (-1.769, 68.4361)
  arc A0 (1.769, 68.4361) -> (-1.769, 68.4361) centre (0, 44) ccw
  line L4 (1.769, 68.4361) -> (17.6369, 68.4361)
  line L5 (17.6369, 68.4361) -> (17.6369, 88.6361)
  line L6 (17.6369, 88.6361) -> (-0.3631, 88.6361)
  line L7 (-44.4367, 43.1482) -> (-45.9367, 43.1482)
  line L8 (-45.9367, 43.1482) -> (-45.9367, 28.1482)
  line L9 (-45.9367, 28.1482) -> (-24.4367, 28.1482)
  line L10 (-24.4367, 28.1482) -> (-24.4367, 42.2395)
  arc A1 (-24.4367, 45.7605) -> (-24.4367, 42.2395) centre (0, 44) ccw
  line L11 (-24.4367, 45.7605) -> (-24.4367, 61.1482)
  line L12 (-24.4367, 61.1482) -> (-44.4367, 61.1482)
  line L13 (-44.4367, 61.1482) -> (-44.4367, 43.1482)
  line L14 (44.6719, 44.6827) -> (46.1719, 44.6827)
  line L15 (46.1719, 44.6827) -> (46.1719, 59.6827)
  line L16 (46.1719, 59.6827) -> (24.6719, 59.6827)
  line L17 (24.6719, 59.6827) -> (24.6719, 26.6827)
  line L18 (24.6719, 26.6827) -> (44.6719, 26.6827)
  line L19 (44.6719, 26.6827) -> (44.6719, 44.6827)
  circle A2 centre (0, 44) radius 15
  arc A3 (-4.6879, 21.9938) -> (-8.5109, 23.1718) centre (0, 44) ccw
  line L20 (-8.5109, 23.1718) -> (-9.0924, 21.2496)
  arc A4 (-9.0924, 21.2496) -> (-5.2376, 20.0664) centre (0, 44) ccw
  line L21 (-5.2376, 20.0664) -> (-4.6879, 21.9938)
  circle A5 centre (-18.1776, 19.3047) radius 4
  circle A6 centre (0.3852, 13.3299) radius 4
  circle A7 centre (18.5396, 19.1937) radius 4
  spline S0 degree 3 poles (63.7288, -20.6496) (65.2154, -19.1571) (66.4944, -17.4924) (68.7649, -13.8113) (69.7272, -11.7971) (72.306, -5.1569) (73.3907, -0.0925) (75.6271, 15.3765) (75.7031, 27.5848) (75.699, 43.6773) (75.7004, 47.2431) (75.6988, 60.0806) (75.6375, 69.5938) (74.6239, 81.2948) (74.2612, 84.3857) (72.74, 93.4567) (71.2848, 98.4205) (67.8979, 105.5132) (66.0773, 108.2918) (63.7288, 110.6496) knots -10.519874 -10.519874 -10.519874 -10.519874 -10.011452 -10.011452 -9.47587 -9.47587 -8.291225 -8.291225 -5.698061 -5.698061 -4.959882 -4.959882 -3.040546 -3.040546 -2.359855 -2.359855 -0.998381 -0.998381 0 0 0 0
  spline S1 degree 3 poles (63.7288, 110.6496) (62.1905, 112.1941) (60.4712, 113.5126) (56.6623, 115.8204) (54.5873, 116.7763) (47.7619, 119.2836) (42.5636, 120.2566) (26.7377, 122.1296) (14.3763, 121.8814) (-0.8933, 121.852) (-3.33, 121.8604) (-18.2109, 121.9208) (-30.8122, 122.029) (-47.118, 119.3949) (-51.7925, 118.0573) (-58.6783, 114.7885) (-61.4038, 112.9839) (-63.7288, 110.6496) knots -8.686827 -8.686827 -8.686827 -8.686827 -8.311039 -8.311039 -7.919015 -7.919015 -7.056807 -7.056807 -5.169739 -5.169739 -4.779276 -4.779276 -2.288129 -2.288129 -0.98839 -0.98839 0 0 0 0
  spline S2 degree 3 poles (-63.7288, 110.6496) (-65.2154, 109.1571) (-66.4944, 107.4924) (-68.7649, 103.8113) (-69.7272, 101.7971) (-72.306, 95.1569) (-73.3907, 90.0925) (-75.6271, 74.6235) (-75.7031, 62.4152) (-75.699, 46.3227) (-75.7004, 42.7569) (-75.6988, 29.9194) (-75.6375, 20.4062) (-74.6239, 8.7052) (-74.2612, 5.6143) (-72.74, -3.4567) (-71.2848, -8.4205) (-67.8979, -15.5132) (-66.0773, -18.2918) (-63.7288, -20.6496) knots -10.519874 -10.519874 -10.519874 -10.519874 -10.011452 -10.011452 -9.47587 -9.47587 -8.291225 -8.291225 -5.698061 -5.698061 -4.959882 -4.959882 -3.040546 -3.040546 -2.359855 -2.359855 -0.998381 -0.998381 0 0 0 0
  spline S3 degree 3 poles (-63.7288, -20.6496) (-62.1905, -22.1941) (-60.4712, -23.5126) (-56.6623, -25.8204) (-54.5873, -26.7763) (-47.7619, -29.2836) (-42.5636, -30.2566) (-26.7377, -32.1296) (-14.3763, -31.8814) (0.8933, -31.852) (3.33, -31.8604) (18.2109, -31.9208) (30.8122, -32.029) (47.118, -29.3949) (51.7925, -28.0573) (58.6783, -24.7885) (61.4038, -22.9839) (63.7288, -20.6496) knots -8.686827 -8.686827 -8.686827 -8.686827 -8.311039 -8.311039 -7.919015 -7.919015 -7.056807 -7.056807 -5.169739 -5.169739 -4.779276 -4.779276 -2.288129 -2.288129 -0.98839 -0.98839 0 0 0 0
  circle A8 centre (0, 44) radius 53.6982
  circle A9 centre (0, 44) radius 53.6982
  circle A10 centre (0, 44) radius 56.6982
  spline S4 degree 3 poles (60.8964, -17.8241) (58.8973, -19.8313) (56.5396, -21.3745) (50.4677, -24.2575) (46.1642, -25.4974) (30.5108, -28.0252) (18.0981, -27.9176) (-0.0843, -27.8427) (-5.5511, -27.8739) (-21.6685, -27.9102) (-32.0285, -27.783) (-44.8034, -25.7159) (-48.87, -24.7598) (-56.0513, -21.7676) (-58.7748, -19.9542) (-60.8964, -17.8241) knots 0 0 0 0 0.849877 0.849877 2.022254 2.022254 4.325903 4.325903 5.316274 5.316274 7.245816 7.245816 8.091874 8.091874 8.906634 8.906634 8.906634 8.906634
  spline S5 degree 3 poles (-60.8964, -17.8241) (-61.8377, -16.879) (-62.6925, -15.9118) (-65.6973, -11.3257) (-67.1217, -7.9014) (-70.2367, 3.1835) (-71.0536, 11.7242) (-71.7206, 27.827) (-71.6855, 35.5544) (-71.6939, 53.5856) (-71.7138, 59.5894) (-71.2837, 75.0773) (-70.6326, 84.055) (-68.0279, 95.0002) (-66.9445, 98.3854) (-63.7701, 104.6689) (-62.239, 106.4761) (-60.8964, 107.8241) knots 0.109418 0.109418 0.109418 0.109418 0.531767 0.531767 1.245442 1.245442 2.56245 2.56245 3.70873 3.70873 4.467113 4.467113 5.530788 5.530788 5.990112 5.990112 6.476468 6.476468 6.476468 6.476468
  spline S6 degree 3 poles (-60.8964, 107.8241) (-58.8973, 109.8313) (-56.5396, 111.3745) (-50.4677, 114.2575) (-46.1642, 115.4974) (-30.5108, 118.0252) (-18.0981, 117.9176) (0.0843, 117.8427) (5.5511, 117.8739) (21.6685, 117.9102) (32.0285, 117.783) (44.8034, 115.7159) (48.87, 114.7598) (56.0513, 111.7676) (58.7748, 109.9542) (60.8964, 107.8241) knots 0 0 0 0 0.849877 0.849877 2.022254 2.022254 4.325903 4.325903 5.316274 5.316274 7.245816 7.245816 8.091874 8.091874 8.906634 8.906634 8.906634 8.906634
  spline S7 degree 3 poles (60.8964, 107.8241) (61.8377, 106.879) (62.6925, 105.9118) (65.6973, 101.3257) (67.1217, 97.9014) (70.2367, 86.8165) (71.0536, 78.2758) (71.7206, 62.173) (71.6855, 54.4456) (71.6939, 36.4144) (71.7138, 30.4106) (71.2837, 14.9227) (70.6326, 5.945) (68.0279, -5.0002) (66.9445, -8.3854) (63.7701, -14.6689) (62.239, -16.4761) (60.8964, -17.8241) knots 0.109418 0.109418 0.109418 0.109418 0.531767 0.531767 1.245442 1.245442 2.56245 2.56245 3.70873 3.70873 4.467113 4.467113 5.530788 5.530788 5.990112 5.990112 6.476468 6.476468 6.476468 6.476468
ref_plane "WorkPlane19" through (0, 0, 120) normal (0, 0, 1) x (1, 0, 0)